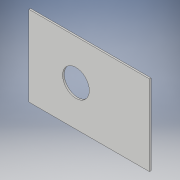
# Autodesk Inventor part: ShooterWall
Saved by Autodesk Inventor 2017 (Build 210142000, 142)
## iProperties
Created: 2016-09-18
Part Number: ShooterWall
Material: Generic
Document SubType Name: Modeling
Designer: Spartacles
Density: 1 g/cm^3
Appearance: Default
Author: Spartacles
Autodesk Inventor part; units mm, degrees
ref_plane "YZ Plane" through (0, 0, 0) normal (1, 0, 0) x (0, 1, 0)
ref_plane "XZ Plane" through (0, 0, 0) normal (0, 1, 0) x (-1, 0, 0)
ref_plane "XY Plane" through (0, 0, 0) normal (0, 0, 1) x (1, 0, 0)
sketch "Sketch1" plane through (0, 0, 0) normal (0, 0, 1) x (1, 0, 0)
  line L0 (0, 0) -> (457.2, 0)
  line L1 (457.2, 0) -> (457.2, 304.8)
  line L2 (457.2, 304.8) -> (0, 304.8)
  line L3 (0, 304.8) -> (0, 0)
  line L4 (0, 254) -> (457.2, 254)
  arc A0 (0.6776, 254) -> (325.1105, 153.4434) centre (178.4776, 254) ccw
  circle A1 centre (178.4776, 152.4) radius 50.8
  line L5 (394.0694, 254) -> (325.1105, 153.4434)
  dimension "d0" = 457.2
  dimension "d1" = 304.8
  dimension "d4" = 101.6
  constraints: 12 end point, 5 point on line, 2 centre point, 2 parallel, 2 perpendicular, 2 point on circle, 1 horizontal, 1 tangent
  measures "d0" distance of L2.end L1.end
  measures "d1" distance of L1.end L0.end
  measures "d4" diameter of A1
sketch "Sketch2" plane through (0, 0, 0) normal (0, 0, 1) x (1, 0, 0)
  point P0 (0, 0)
extrude "Extrusion1" add sketch "Sketch1" along normal blind 6.35
body "Solid1"
